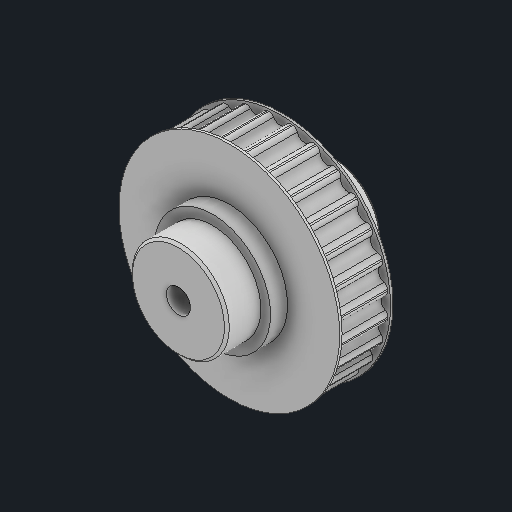
# Autodesk Inventor part: 28teeth_gear
Saved by Autodesk Inventor 2026 (Build 300175000, 175)
## iProperties
Created: 2025-07-14
Part Number: 28teeth_gear
Material: Generic
Document SubType Name: Modeling
Designer: User
Density: 1 g/cm^3
Appearance: Default
Author: User
Autodesk Inventor part; units mm, degrees
ref_plane "YZ Plane" through (0, 0, 0) normal (1, 0, 0) x (0, 1, 0)
ref_plane "XZ Plane" through (0, 0, 0) normal (0, 1, 0) x (-1, 0, 0)
ref_plane "XY Plane" through (0, 0, 0) normal (0, 0, 1) x (1, 0, 0)
sketch "Sketch1" plane through (0, 0, 0) normal (0, 0, 1) x (1, 0, 0)
  circle A0 centre (0, 0) radius 22.3
  dimension "d0" = 44.6
  constraints: 1 centre point, 1 coincident
  measures "d0" diameter of A0
extrude "Extrusion1" add sketch "Sketch1" along normal blind 10
sketch "Sketch2" plane through (0, 0, 10) normal (0, 0, 1) x (1, 0, 0)
  circle A0 centre (0, 0) radius 22.3 construction
  circle A1 centre (0, 0) radius 20.8 construction
  circle A2 centre (0, 22.3) radius 1.5
  circle A3 centre (0, 0) radius 20.8 construction
  circle A4 centre (-4.9622, 21.7409) radius 1.5
  circle A5 centre (0, 0) radius 20.8 construction
  circle A6 centre (-9.6756, 20.0916) radius 1.5
  circle A7 centre (0, 0) radius 20.8 construction
  circle A8 centre (-13.9038, 17.4348) radius 1.5
  circle A9 centre (0, 0) radius 20.8 construction
  circle A10 centre (-17.4348, 13.9038) radius 1.5
  circle A11 centre (0, 0) radius 20.8 construction
  circle A12 centre (-20.0916, 9.6756) radius 1.5
  circle A13 centre (0, 0) radius 20.8 construction
  circle A14 centre (-21.7409, 4.9622) radius 1.5
  circle A15 centre (0, 0) radius 20.8 construction
  circle A16 centre (-22.3, 0) radius 1.5
  circle A17 centre (0, 0) radius 20.8 construction
  circle A18 centre (-21.7409, -4.9622) radius 1.5
  circle A19 centre (0, 0) radius 20.8 construction
  circle A20 centre (-20.0916, -9.6756) radius 1.5
  circle A21 centre (0, 0) radius 20.8 construction
  circle A22 centre (-17.4348, -13.9038) radius 1.5
  circle A23 centre (0, 0) radius 20.8 construction
  circle A24 centre (-13.9038, -17.4348) radius 1.5
  circle A25 centre (0, 0) radius 20.8 construction
  circle A26 centre (-9.6756, -20.0916) radius 1.5
  circle A27 centre (0, 0) radius 20.8 construction
  circle A28 centre (-4.9622, -21.7409) radius 1.5
  circle A29 centre (0, 0) radius 20.8 construction
  circle A30 centre (0, -22.3) radius 1.5
  circle A31 centre (0, 0) radius 20.8 construction
  circle A32 centre (4.9622, -21.7409) radius 1.5
  circle A33 centre (0, 0) radius 20.8 construction
  circle A34 centre (9.6756, -20.0916) radius 1.5
  circle A35 centre (0, 0) radius 20.8 construction
  circle A36 centre (13.9038, -17.4348) radius 1.5
  circle A37 centre (0, 0) radius 20.8 construction
  circle A38 centre (17.4348, -13.9038) radius 1.5
  circle A39 centre (0, 0) radius 20.8 construction
  circle A40 centre (20.0916, -9.6756) radius 1.5
  circle A41 centre (0, 0) radius 20.8 construction
  circle A42 centre (21.7409, -4.9622) radius 1.5
  circle A43 centre (0, 0) radius 20.8 construction
  circle A44 centre (22.3, 0) radius 1.5
  circle A45 centre (0, 0) radius 20.8 construction
  circle A46 centre (21.7409, 4.9622) radius 1.5
  circle A47 centre (0, 0) radius 20.8 construction
  circle A48 centre (20.0916, 9.6756) radius 1.5
  circle A49 centre (0, 0) radius 20.8 construction
  circle A50 centre (17.4348, 13.9038) radius 1.5
  circle A51 centre (0, 0) radius 20.8 construction
  circle A52 centre (13.9038, 17.4348) radius 1.5
  circle A53 centre (0, 0) radius 20.8 construction
  circle A54 centre (9.6756, 20.0916) radius 1.5
  circle A55 centre (0, 0) radius 20.8 construction
  circle A56 centre (4.9622, 21.7409) radius 1.5
  dimension "d3" = 1.5
  dimension "d6" = 360
  constraints: 56 centre point, 1 tangent, 1 vertical alignment, 114 other
extrude "Extrusion2" cut sketch "Sketch2" against normal blind 10
fillet "Fillet1" radius 1 56 edges at (8.303, 20.6966, 5) (11.0044, 19.3957, 5) (3.4894, 22.0253, 5) (6.4126, 21.3581, 5) (12.7003, 18.3301, 5) (15.0445, 16.4607, 5) (16.4607, 15.0445, 5) (18.3301, 12.7003, 5) (19.3957, 11.0044, 5) (20.6966, 8.303, 5) (22.0253, 3.4894, 5) (21.3581, 6.4126, 5) (22.2496, 1.4992, 5) (22.2496, -1.4992, 5) (22.0253, -3.4894, 5) (21.3581, -6.4126, 5) (20.6966, -8.303, 5) (19.3957, -11.0044, 5) (18.3301, -12.7003, 5) (16.4607, -15.0445, 5) (15.0445, -16.4607, 5) (12.7003, -18.3301, 5) (11.0044, -19.3957, 5) (8.303, -20.6966, 5) (6.4126, -21.3581, 5) (3.4894, -22.0253, 5) (1.4992, -22.2496, 5) (-1.4992, -22.2496, 5) (-3.4894, -22.0253, 5) (-6.4126, -21.3581, 5) (-8.303, -20.6966, 5) (-11.0044, -19.3957, 5) (-12.7003, -18.3301, 5) (-15.0445, -16.4607, 5) (-16.4607, -15.0445, 5) (-18.3301, -12.7003, 5) (-19.3957, -11.0044, 5) (-20.6966, -8.303, 5) (-21.3581, -6.4126, 5) (-22.0253, -3.4894, 5) (-22.2496, -1.4992, 5) (-22.2496, 1.4992, 5) (-22.0253, 3.4894, 5) (-21.3581, 6.4126, 5) (-20.6966, 8.303, 5) (-19.3957, 11.0044, 5) (-18.3301, 12.7003, 5) (-16.4607, 15.0445, 5) (-15.0445, 16.4607, 5) (-12.7003, 18.3301, 5) (-11.0044, 19.3957, 5) (-8.303, 20.6966, 5) (-6.4126, 21.3581, 5) (-3.4894, 22.0253, 5) (-1.4992, 22.2496, 5) (1.4992, 22.2496, 5)
sketch "Sketch3" plane through (0, 0, 0) normal (0, 0, -1) x (-1, 0, 0)
  circle A0 centre (0, 0) radius 22.75
  dimension "d11" = 45.5
  constraints: 1 centre point, 1 coincident
  measures "d11" diameter of A0
extrude "Extrusion3" add sketch "Sketch3" along normal blind 0.5
sketch "Sketch4" plane through (0, 0, 10) normal (0, 0, 1) x (1, 0, 0)
  circle A0 centre (0, 0) radius 22.75
  dimension "d14" = 45.5
  constraints: 1 centre point, 1 coincident
  measures "d14" diameter of A0
extrude "Extrusion4" add sketch "Sketch4" along normal blind 0.5
sketch "Sketch5" plane through (0, 0, 10.5) normal (0, 0, 1) x (1, 0, 0)
  circle A0 centre (0, 0) radius 12
  dimension "d17" = 24
  constraints: 1 centre point, 1 coincident
  measures "d17" diameter of A0
extrude "Extrusion5" add sketch "Sketch5" along normal blind 3.5
sketch "Sketch6" plane through (0, 0, 14) normal (0, 0, 1) x (1, 0, 0)
  circle A0 centre (0, 0) radius 10
  dimension "d20" = 20
  constraints: 1 centre point, 1 coincident
  measures "d20" diameter of A0
extrude "Extrusion6" add sketch "Sketch6" along normal blind 7
sketch "Sketch7" plane through (0, 0, -0.5) normal (0, 0, -1) x (-1, 0, 0)
  circle A0 centre (0, 0) radius 12
  dimension "d23" = 24
  constraints: 1 centre point, 1 coincident
  measures "d23" diameter of A0
extrude "Extrusion7" add sketch "Sketch7" along normal blind 3.5
sketch "Sketch8" plane through (0, 0, -4) normal (0, 0, -1) x (-1, 0, 0)
  circle A0 centre (0, 0) radius 10
  dimension "d26" = 20
  constraints: 1 centre point, 1 coincident
  measures "d26" diameter of A0
extrude "Extrusion8" add sketch "Sketch8" along normal blind 7
sketch "Sketch9" plane through (0, 0, 21) normal (0, 0, 1) x (1, 0, 0)
  circle A0 centre (0, 0) radius 2.5
  dimension "d29" = 5
  constraints: 1 centre point, 1 coincident
  measures "d29" diameter of A0
extrude "Extrusion9" cut sketch "Sketch9" against normal blind 43.3375
chamfer "Chamfer1" distance 0.5 angle 45 2 edges at (10, 0, -11) (-10, 0, 21)
body "Solid1"
